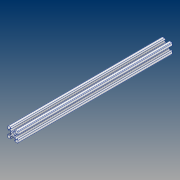
# Autodesk Inventor part: 20x20x300
Saved by Autodesk Inventor 2021 (Build 250183000, 183)
## iProperties
Created: 2020-04-01
Part Number: 20x20x300
Material: Aluminum 6061
Document SubType Name: Modeling
Designer: Sunoj
Density: 2.7 g/cm^3
Appearance: Aluminum - Flat
Author: Sunoj
Autodesk Inventor part; units mm, degrees
ref_plane "YZ Plane" through (0, 0, 0) normal (1, 0, 0) x (0, 1, 0)
ref_plane "XZ Plane" through (0, 0, 0) normal (0, 1, 0) x (-1, 0, 0)
ref_plane "XY Plane" through (0, 0, 0) normal (0, 0, 1) x (1, 0, 0)
sketch "Sketch1" plane through (0, 0, 0) normal (0, 0, 1) x (1, 0, 0)
  line L0 (-14, 8.7) -> (-14, 6.0607)
  line L1 (-14, 8.7) -> (-14, 6.0607)
  line L2 (-14, 6.0607) -> (-16.5607, 3.5)
  line L3 (-14, 6.0607) -> (-16.5607, 3.5)
  line L4 (-16.5607, 3.5) -> (-18.2, 3.5)
  line L5 (-16.5607, 3.5) -> (-18.2, 3.5)
  line L6 (-18.2, 3.5) -> (-18.2, 6)
  line L7 (-18.2, 3.5) -> (-18.2, 6)
  line L8 (-20, 4.2) -> (-20, 0)
  line L9 (-18.2, 6) -> (-20, 4.2)
  line L10 (-20, 4.2) -> (-20, 0)
  line L11 (-19, -1) -> (-14.8, -1)
  line L12 (-19, -1) -> (-14.8, -1)
  line L13 (-14.8, -1) -> (-13, 0.8)
  line L14 (-14.8, -1) -> (-13, 0.8)
  line L15 (-15.5, 0.8) -> (-15.5, 2.4393)
  line L16 (-13, 0.8) -> (-15.5, 0.8)
  line L17 (-15.5, 0.8) -> (-15.5, 2.4393)
  line L18 (-12.9393, 5) -> (-10.3, 5)
  line L19 (-15.5, 2.4393) -> (-12.9393, 5)
  line L20 (-12.9393, 5) -> (-10.3, 5)
  line L21 (-10, 5.3) -> (-9.7, 5)
  line L22 (-10.3, 5) -> (-10, 5.3)
  line L23 (-13.7, 9) -> (-14, 8.7)
  line L24 (-13.7, 9) -> (-14, 8.7)
  line L25 (-10, 9) -> (-10, 10.0607)
  circle A0 centre (-10, 9) radius 2.5
  arc A1 (-20, 0) -> (-19, -1) centre (-19, 0) ccw
  arc A2 (-20, 0) -> (-19, -1) centre (-19, 0) ccw
  line L26 (-7.0607, 5) -> (-4.5, 2.4393)
  line L27 (-4.5, 2.4393) -> (-4.5, 0.8)
  line L28 (-4.5, 0.8) -> (-7, 0.8)
  line L29 (-7, 0.8) -> (-5.2, -1)
  line L30 (-3.4393, 3.5) -> (-6, 6.0607)
  line L31 (-1.8, 6) -> (-1.8, 3.5)
  line L32 (-1.8, 3.5) -> (-3.4393, 3.5)
  line L33 (0, 4.2) -> (-1.8, 6)
  line L34 (-5.2, -1) -> (-1, -1)
  line L35 (0, 0) -> (0, 4.2)
  arc A3 (-1, -1) -> (0, 0) centre (-1, 0) ccw
  line L36 (-9.7, 5) -> (-7.0607, 5)
  line L37 (-6, 6.0607) -> (-6, 8.7)
  line L38 (-6, 8.7) -> (-6.3, 9)
  line L39 (-10, 5.3) -> (-9.7, 5)
  line L40 (-6, 11.9393) -> (-3.4393, 14.5)
  line L41 (-3.4393, 14.5) -> (-1.8, 14.5)
  line L42 (-1.8, 14.5) -> (-1.8, 12)
  line L43 (-1.8, 12) -> (0, 13.8)
  line L44 (-4.5, 15.5607) -> (-7.0607, 13)
  line L45 (-7, 17.2) -> (-4.5, 17.2)
  line L46 (-4.5, 17.2) -> (-4.5, 15.5607)
  line L47 (-5.2, 19) -> (-7, 17.2)
  line L48 (0, 13.8) -> (0, 18)
  line L49 (-1, 19) -> (-5.2, 19)
  arc A4 (0, 18) -> (-1, 19) centre (-1, 18) ccw
  line L50 (-6, 9.3) -> (-6, 11.9393)
  line L51 (-7.0607, 13) -> (-9.7, 13)
  line L52 (-9.7, 13) -> (-10, 12.7)
  line L53 (-6.3, 9) -> (-6, 9.3)
  line L54 (-12.9393, 13) -> (-15.5, 15.5607)
  line L55 (-15.5, 15.5607) -> (-15.5, 17.2)
  line L56 (-15.5, 17.2) -> (-13, 17.2)
  line L57 (-13, 17.2) -> (-14.8, 19)
  line L58 (-16.5607, 14.5) -> (-14, 11.9393)
  line L59 (-18.2, 12) -> (-18.2, 14.5)
  line L60 (-18.2, 14.5) -> (-16.5607, 14.5)
  line L61 (-20, 13.8) -> (-18.2, 12)
  line L62 (-14.8, 19) -> (-19, 19)
  line L63 (-20, 18) -> (-20, 13.8)
  arc A5 (-19, 19) -> (-20, 18) centre (-19, 18) ccw
  line L64 (-10.3, 13) -> (-12.9393, 13)
  line L65 (-14, 11.9393) -> (-14, 9.3)
  line L66 (-14, 9.3) -> (-13.7, 9)
  line L67 (-10, 12.7) -> (-10.3, 13)
  point P0 (0, 0)
  point P1 (-1, 0)
  point P2 (-1, 18)
  point P3 (-19, 18)
  dimension "d2" = 360
  constraints: 136 end point, 10 point on circle, 9 collinear, 6 centre point, 3 parallel, 2 perpendicular, 1 coincident, 1 concentric, 1 vertical, 133 other
extrude "Extrusion1" add sketch "Sketch1" along normal blind 300
body "Solid1"
